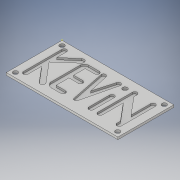
# Autodesk Inventor part: klam final
Saved by Autodesk Inventor 2017 (Build 210142000, 142)
## iProperties
Created: 2016-09-22
Part Number: klam final
Material: Generic
Document SubType Name: Modeling
Designer: vslabsal
Density: 1 g/cm^3
Appearance: Default
Author: vslabsal
Autodesk Inventor part; units mm, degrees
ref_plane "YZ Plane" through (0, 0, 0) normal (1, 0, 0) x (0, 1, 0)
ref_plane "XZ Plane" through (0, 0, 0) normal (0, 1, 0) x (-1, 0, 0)
ref_plane "XY Plane" through (0, 0, 0) normal (0, 0, 1) x (1, 0, 0)
sketch "Sketch1" plane through (0, 0, 0) normal (0, 1, 0) x (-1, 0, 0)
  line L0 (0, 0) -> (-152.4, 0)
  line L1 (-152.4, 0) -> (-152.4, 76.2)
  line L2 (-152.4, 76.2) -> (0, 76.2)
  line L3 (0, 76.2) -> (0, 0)
  constraints: 8 end point, 2 parallel, 1 horizontal, 1 perpendicular
extrude "Extrusion1" add sketch "Sketch1" along normal blind 3.175
sketch "Sketch2" plane through (0, 3.175, 0) normal (0, 1, 0) x (1, 0, 0)
  point P0 (0, 0)
sketch "Sketch3" plane through (0, 3.175, 0) normal (0, 1, 0) x (1, 0, 0)
  point P0 (0, 0)
sketch "Sketch4" plane through (0, 3.175, 0) normal (0, 1, 0) x (1, 0, 0)
  circle A0 centre (6.35, -6.35) radius 3.175
  circle A1 centre (6.35, -69.9426) radius 3.175
  circle A2 centre (145.8663, -69.9426) radius 3.175
  circle A3 centre (145.8663, -6.35) radius 3.175
  point P0 (0, 0)
  constraints: 4 centre point
hole "Hole1" at (6.35, 3.175, 6.35) at (6.35, 3.175, 69.9426) at (145.8663, 3.175, 69.9426) at (145.8663, 3.175, 6.35) direction (0, -1, 0) diameter 6.35 end through all
sketch "Sketch5" plane through (0, 3.175, 0) normal (0, 1, 0) x (1, 0, 0)
  line L0 (10.5157, -11.0499) -> (10.5124, -63.5081)
  arc A0 (16.7318, -11.0499) -> (10.5157, -11.0499) centre (13.6238, -10.7421) ccw
  arc A1 (10.5124, -63.5081) -> (16.7351, -63.5081) centre (13.6238, -63.5083) ccw
  line L1 (16.7318, -24.057) -> (34.8293, -8.3141)
  line L2 (16.7369, -34.4606) -> (39.8985, -14.1414)
  line L3 (16.7369, -34.4606) -> (39.3705, -61.398)
  line L4 (34.3364, -65.6278) -> (16.7351, -44.6796)
  line L5 (16.7318, -11.0499) -> (16.7318, -24.057)
  line L6 (16.7351, -44.6796) -> (16.7351, -63.5081)
  arc A2 (39.8985, -14.1414) -> (34.8293, -8.3141) centre (37.3639, -11.2278) ccw
  arc A3 (34.3364, -65.6278) -> (39.3705, -61.398) centre (36.8535, -63.5129) ccw
  arc A4 (61.8542, -17.5534) -> (61.8542, -11.2278) centre (61.8542, -14.3906) ccw
  arc A5 (61.8927, -39.7278) -> (61.8542, -33.4021) centre (61.8734, -36.5649) ccw
  arc A6 (61.8542, -63.5501) -> (61.8542, -57.2244) centre (61.8542, -60.3873) ccw
  line L7 (61.8542, -11.2278) -> (47.9378, -11.2278)
  line L8 (49.1549, -33.4021) -> (49.1549, -17.5534)
  line L9 (49.1549, -39.7278) -> (49.1549, -57.2244)
  line L10 (61.8542, -57.2244) -> (49.1549, -57.2244)
  line L11 (61.8927, -39.7278) -> (49.1549, -39.7278)
  line L12 (61.8542, -17.5534) -> (49.1549, -17.5534)
  line L13 (49.1549, -33.4021) -> (61.8542, -33.4021)
  arc A7 (47.9378, -11.2278) -> (41.5878, -16.1855) centre (47.2856, -16.9379) ccw
  line L14 (41.5878, -16.1855) -> (41.5878, -57.5593)
  line L15 (49.1549, -63.5501) -> (61.8542, -63.5501)
  arc A8 (41.5878, -57.5593) -> (49.1549, -63.5501) centre (49.1549, -55.7757) ccw
  line L16 (67.0028, -13.2236) -> (76.6357, -60.4074)
  line L17 (93.2217, -13.986) -> (81.9862, -60.5027)
  line L18 (73.3373, -13.1484) -> (79.3224, -40.4995)
  line L19 (79.3224, -40.4995) -> (87.3283, -12.4343)
  arc A9 (73.3373, -13.1484) -> (67.0028, -13.2236) centre (70.1778, -13.8398) ccw
  arc A10 (93.2217, -13.986) -> (87.3283, -12.4343) centre (90.2592, -13.2704) ccw
  arc A11 (76.6357, -60.4074) -> (81.9862, -60.5027) centre (79.3216, -59.8591) ccw
  circle A12 centre (100.2447, -14.3906) radius 3.175
  line L20 (97.0697, -32.199) -> (97.0697, -60.5027)
  line L21 (103.4197, -32.199) -> (103.4197, -60.5027)
  arc A13 (97.0697, -60.5027) -> (103.4197, -60.5027) centre (100.2447, -60.5027) ccw
  arc A14 (103.4197, -32.199) -> (97.0697, -32.199) centre (100.2447, -32.199) ccw
  line L22 (109.3457, -13.3836) -> (109.3457, -60.5027)
  line L23 (141.7333, -14.3906) -> (141.7333, -60.5027)
  arc A15 (109.3457, -60.5027) -> (115.6957, -60.5027) centre (112.5207, -60.5027) ccw
  arc A16 (115.6957, -13.3836) -> (109.3457, -13.3836) centre (112.5207, -13.3836) ccw
  arc A17 (141.7333, -14.3906) -> (135.3833, -14.3906) centre (138.5583, -14.3906) ccw
  arc A18 (135.3833, -60.5027) -> (141.7333, -60.5027) centre (138.5583, -60.5027) ccw
  line L24 (115.6957, -17.5656) -> (135.3833, -41.317)
  line L25 (115.6957, -32.199) -> (135.3833, -55.7757)
  line L26 (135.3833, -14.3906) -> (135.3833, -41.317)
  line L27 (135.3833, -55.7757) -> (135.3833, -60.5027)
  line L28 (115.6957, -32.199) -> (115.6957, -60.5027)
  line L29 (115.6957, -17.5656) -> (115.6957, -13.3836)
  point P0 (0, 0)
  constraints: 60 end point, 36 point on circle, 19 centre point, 16 tangent, 4 horizontal, 3 parallel, 3 point on line, 3 vertical, 1 collinear, 1 perpendicular
sketch "Sketch6" plane through (0, 3.175, 0) normal (0, 1, 0) x (1, 0, 0)
  point P0 (0, 0)
extrude "Extrusion2" cut sketch "Sketch5" against normal blind 2.54
body "Solid1"
